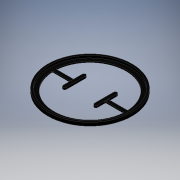
# Autodesk Inventor part: Bumper_modified
Saved by Autodesk Inventor 2016 (Build 200138000, 138)
## iProperties
Created: 2016-07-25
Part Number: Bumper_modified
Material: Plastique ABS
Document SubType Name: Modeling
Designer: tmonglon
Density: 1.06 g/cm^3
Appearance: Lisse - Noir
Author: tmonglon
Autodesk Inventor part; units mm, degrees
ref_plane "YZ Plane" through (0, 0, 0) normal (1, 0, 0) x (0, 1, 0)
ref_plane "XZ Plane" through (0, 0, 0) normal (0, 1, 0) x (-1, 0, 0)
ref_plane "XY Plane" through (0, 0, 0) normal (0, 0, 1) x (1, 0, 0)
sketch "Esquisse1" plane through (0, 0, 0) normal (0, 0, 1) x (1, 0, 0)
  circle A0 centre (0, 0) radius 63
  circle A1 centre (0, 0) radius 60
  circle A2 centre (0, 0) radius 54
  line L0 (-25.9421, 2.5) -> (-53.9421, 2.5)
  line L1 (-25.9421, -2.5) -> (-53.9421, -2.5)
  line L2 (-20.9421, 0) -> (-20.9421, 14.5)
  line L3 (-25.9421, 14.5) -> (-25.9421, 2.5)
  line L4 (-20.9421, 0) -> (-20.9421, -14.5)
  line L5 (-25.9421, -14.5) -> (-25.9421, 2.5)
  arc A3 (-25.9421, -14.5) -> (-20.9421, -14.5) centre (-23.4421, -14.5) ccw
  arc A4 (-20.9421, 14.5) -> (-25.9421, 14.5) centre (-23.4421, 14.5) ccw
  line L6 (0, 0) -> (0, 11.8583)
  line L7 (25.9421, 2.5) -> (53.9421, 2.5)
  line L8 (25.9421, -2.5) -> (53.9421, -2.5)
  line L9 (20.9421, 0) -> (20.9421, 14.5)
  line L10 (25.9421, 14.5) -> (25.9421, 2.5)
  line L11 (20.9421, 0) -> (20.9421, -14.5)
  line L12 (25.9421, -14.5) -> (25.9421, 14.5)
  arc A5 (20.9421, -14.5) -> (25.9421, -14.5) centre (23.4421, -14.5) ccw
  arc A6 (25.9421, 14.5) -> (20.9421, 14.5) centre (23.4421, 14.5) ccw
  line L13 (25.9421, 2.5) -> (56.5559, 2.5)
  line L14 (56.5559, 2.5) -> (56.5559, -2.5)
  line L15 (56.5559, -2.5) -> (25.9421, -2.5)
  line L16 (25.9421, -2.5) -> (25.9421, 2.5)
  dimension "d0" = 126
  dimension "d1" = 120
  dimension "d2" = 108
  dimension "d3" = 28
  dimension "d6" = 14.5
  dimension "d8" = 5
  constraints: 34 end point, 11 point on circle, 11 symmetric about line, 7 centre point, 6 point on line, 4 parallel, 1 coincident, 1 horizontal, 1 perpendicular, 1 vertical, 2 other
  measures "d0" diameter of A0
  measures "d1" diameter of A1
  measures "d2" diameter of A2
  measures "d3" distance of L0.start L0.end
  measures "d6" distance of L2.start L2.end
  measures "d8" distance of L4.end L5.start
extrude "Extrusion1" add sketch "Esquisse1" along normal blind 5 contours A0
extrude "Extrusion2" add sketch "Esquisse1" along normal blind 1.7 contours A1 | A2 L8 L12 L7 | A2 L13 L14 L15 | L0 L5 L1 A2
sketch "Esquisse3" plane through (0, 0, 0) normal (0, 0, -1) x (-1, 0, 0)
  line L0 (20.9421, 0) -> (20.9421, 14.5) projected
  line L1 (20.9421, 0) -> (20.9421, -14.5) projected
  arc A0 (20.9421, -14.5) -> (25.9421, -14.5) centre (23.4421, -14.5) ccw projected
  line L2 (25.9421, -14.5) -> (25.9421, 2.5) projected
  line L3 (25.9421, 14.5) -> (25.9421, 2.5) projected
  arc A1 (25.9421, 14.5) -> (20.9421, 14.5) centre (23.4421, 14.5) ccw projected
  arc A2 (-20.9421, 14.5) -> (-25.9421, 14.5) centre (-23.4421, 14.5) ccw projected
  line L4 (-25.9421, 14.5) -> (-25.9421, 2.5) projected
  line L5 (-25.9421, -14.5) -> (-25.9421, 14.5) projected
  arc A3 (-25.9421, -14.5) -> (-20.9421, -14.5) centre (-23.4421, -14.5) ccw projected
  line L6 (-20.9421, 0) -> (-20.9421, -14.5) projected
  line L7 (-20.9421, 0) -> (-20.9421, 14.5) projected
  point P0 (0, 0)
extrude "Extrusion3" add sketch "Esquisse3" against normal blind 3
fillet "Congé1" radius 1 3 edges at (25.9421, 0, 1.7) (25.9421, -2.5, 0.85) (25.9421, 2.5, 0.85)
fillet "Congé2" radius 1 3 edges at (-25.9421, 0, 1.7) (-25.9421, -2.5, 0.85) (-25.9421, 2.5, 0.85)
fillet "Congé3" radius 1 4 edges at (53.9421, 2.5, 0.85) (53.9421, -2.5, 0.85) (-53.9421, 2.5, 0.85) (-53.9421, -2.5, 0.85)
